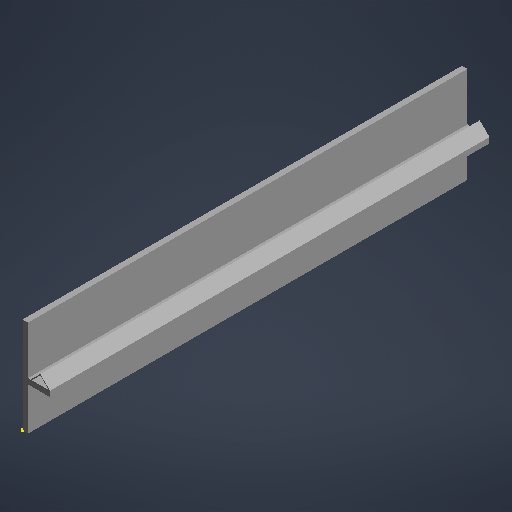
# Autodesk Inventor part: Riel superior
Saved by Autodesk Inventor 2026.2 (Build 302298010, 298A)
## iProperties
Part Number: Riel superior
Material: Generic
Document SubType Name: Modeling
Designer: diego
Appearance: Default
Author: diego
Autodesk Inventor part; units mm, degrees
ref_plane "YZ Plane" through (0, 0, 0) normal (1, 0, 0) x (0, 1, 0)
ref_plane "XZ Plane" through (0, 0, 0) normal (0, 1, 0) x (-1, 0, 0)
ref_plane "XY Plane" through (0, 0, 0) normal (0, 0, 1) x (1, 0, 0)
sketch "Sketch1" plane through (0, 0, 0) normal (1, 0, 0) x (0, 1, 0)
  line L0 (0, 0) -> (350, 0)
  line L1 (350, 0) -> (350, -1600)
  line L2 (350, -1600) -> (0, -1600)
  line L3 (0, -1600) -> (0, 0)
  dimension "d0" = 350
  dimension "d1" = 1600
  constraints: 8 end point, 2 parallel, 1 horizontal, 1 perpendicular
  measures "d0" distance of L1.end L2.end
  measures "d1" distance of L0.end L1.end
extrude "Extrusion1" add sketch "Sketch1" along normal blind 20
sketch "Sketch3" plane through (0, 0, 0) normal (0, 0, 1) x (1, 0, 0)
  point P0 (0, 0)
sketch "Sketch6" plane through (20, 0, 0) normal (1, 0, 0) x (0, 0, -1)
  line L0 (0, 350) -> (0, 0) projected
  line L1 (1600, 0) -> (1600, 350) projected
  line L2 (0, 175) -> (1600, 175)
  line L3 (1600, 175) -> (1600, 155)
  line L4 (1600, 155) -> (0, 155)
  line L5 (0, 155) -> (0, 175)
  point P0 (0, 155)
  dimension "d11" = 20
  constraints: 8 end point, 2 parallel, 1 horizontal, 1 midpoint, 1 perpendicular, 1 point on line
  measures "d11" distance between parallel lines of L4 L2
extrude "Extrusion4" add sketch "Sketch6" along normal blind 80
sketch "Sketch7" plane through (0, 0, 0) normal (0, 0, 1) x (1, 0, 0)
  line L0 (100, 155) -> (100, 175) projected
  line L1 (100, 175) -> (64.6447, 210.3553)
  line L2 (100, 175) -> (150, 175) construction
  line L3 (64.6447, 210.3553) -> (29.2893, 175)
  line L4 (29.2893, 175) -> (33.532, 175)
  line L5 (20, 175) -> (100, 175) projected
  line L6 (33.532, 175) -> (64.6447, 206.1127)
  line L7 (64.6447, 206.1127) -> (95.7574, 175)
  point P0 (0, 0)
  dimension "d14" = 50
  dimension "d15" = 135
  dimension "d16" = 50
  dimension "d18" = 3
  dimension "d19" = 3
  constraints: 12 end point, 2 perpendicular, 2 point on line, 1 equal length, 1 horizontal, 1 parallel
  measures "d14" distance of L0.end L1.end
  measures "d15" angle of L2 L1
  measures "d16" distance of L1.end L3.end
  measures "d18" distance between parallel lines of L1 L7
  measures "d19" distance between parallel lines of L6 L3
extrude "Extrusion5" add sketch "Sketch7" against normal blind 1600 contours L5 L7 L6 L4 L3 L1
body "Solid1"
